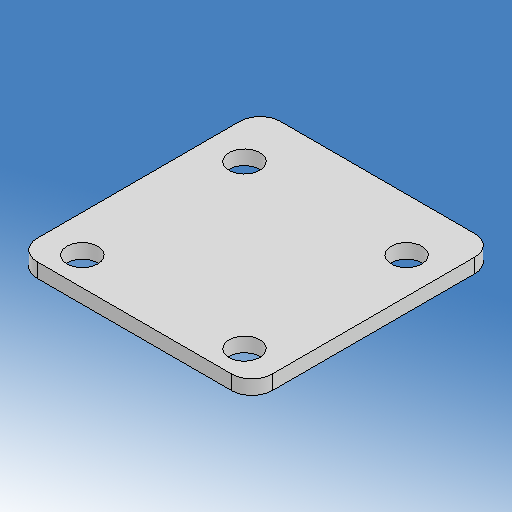
# Autodesk Inventor part: SportGearBox_offsetPlate
Saved by Autodesk Inventor 2025 (Build 290162000, 162)
## iProperties
Created: 2024-06-22
Part Number: SportGearBox_offsetPlate
Material: Generic
Document SubType Name: Modeling
Designer: seene
Density: 1 g/cm^3
Appearance: Default
Author: seene
Autodesk Inventor part; units mm, degrees
ref_plane "YZ Plane" through (0, 0, 0) normal (1, 0, 0) x (0, 1, 0)
ref_plane "XZ Plane" through (0, 0, 0) normal (0, 1, 0) x (-1, 0, 0)
ref_plane "XY Plane" through (0, 0, 0) normal (0, 0, 1) x (1, 0, 0)
sketch "Sketch1" plane through (0, 0, 0) normal (0, 1, 0) x (-1, 0, 0)
  line L0 (0, 0) -> (36.83, 0)
  line L1 (36.83, 0) -> (36.83, -38.1)
  line L2 (36.83, -38.1) -> (0, -38.1)
  line L3 (0, -38.1) -> (0, 0)
  circle A0 centre (31.0167, -4.445) radius 2.413
  circle A1 centre (31.0167, -29.845) radius 2.413
  circle A2 centre (5.6167, -4.445) radius 2.413
  circle A3 centre (5.6167, -29.845) radius 2.413
  dimension "d0" = 4.826
  dimension "d1" = 38.1
  dimension "d2" = 36.83
  dimension "d3" = 4.445
  dimension "d4" = 5.8133
  dimension "d7" = 25.4
  dimension "d10" = 25.4
  constraints: 8 end point, 4 centre point, 2 horizontal, 2 parallel, 1 perpendicular, 1 vertical, 6 other
  measures "d0" diameter of A0
  measures "d1" distance of L0.end L1.end
  measures "d2" distance of L1.end L2.end
  measures "d3" distance from line of A0.centre L0
  measures "d4" distance from line of L1 A0.centre
  measures "d7" distance of A0.centre A1.centre
  measures "d10" distance of A0.centre A2.centre
extrude "Extrusion1" add sketch "Sketch1" along normal blind 2.2561
fillet "Fillet1" radius 3.175 4 edges at (0, 1.1281, 0) (-36.83, 1.1281, 0) (0, 1.1281, -38.1) (-36.83, 1.1281, -38.1)
body "Solid1"
